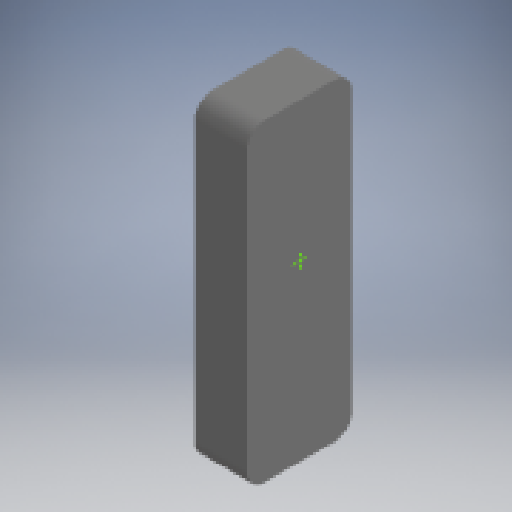
# Autodesk Inventor part: link7
Saved by Autodesk Inventor 2024.1 (Build 281209000, 209)
## iProperties
Created: 2023-09-09
Part Number: link7
Material: Aluminum 6061
Document SubType Name: Modeling
Designer: Camilo
Density: 2.7 g/cm^3
Appearance: Aluminum - Flat
Mass: 7.14896 g
Surface Area: 15.3631 cm^2
Volume: 2.64776 cm^3
Author: Camilo
Autodesk Inventor part; units mm, degrees
ref_plane "YZ Plane" through (0, 0, 0) normal (1, 0, 0) x (0, 1, 0)
ref_plane "XZ Plane" through (0, 0, 0) normal (0, 1, 0) x (-1, 0, 0)
ref_plane "XY Plane" through (0, 0, 0) normal (0, 0, 1) x (1, 0, 0)
sketch "Sketch1" plane through (0, 0, 0) normal (0, 0, 1) x (1, 0, 0)
  line L0 (0, 0) -> (0, 6)
  line L1 (0, 6) -> (-4, 6)
  line L2 (-4, 6) -> (-4, -6)
  line L3 (-4, -6) -> (0, -6)
  line L4 (0, -6) -> (0, 6)
  line L5 (-2, 6) -> (-2, -6)
  line L6 (-2, 6) -> (-2, 3)
  circle A0 centre (-2, 3) radius 1.25
  line L7 (-2, -6) -> (-2, -3)
  circle A1 centre (-2, -3) radius 1.25
  line L8 (0, 6) -> (0, 14)
  line L9 (0, 14) -> (6, 14)
  line L10 (6, 14) -> (6, -22)
  line L11 (6, -22) -> (0, -22)
  line L12 (0, -22) -> (0, 14)
  dimension "d44" = 6
  dimension "d45" = 4
  dimension "d46" = 12
  dimension "d47" = 3
  dimension "d48" = 2.5
  dimension "d49" = 3
  dimension "d50" = 2.5
  dimension "d51" = 8
  dimension "d52" = 6
  dimension "d53" = 36
  constraints: 26 end point, 4 parallel, 2 centre point, 2 coincident, 2 horizontal, 2 midpoint, 2 perpendicular, 2 point on line, 2 vertical
  measures "d44" distance of L0.start L0.end
  measures "d45" distance of L3.end L2.end
  measures "d46" distance of L2.end L1.end
  measures "d47" distance of L5.start L6.end
  measures "d48" diameter of A0
  measures "d49" distance of L5.end L7.end
  measures "d50" diameter of A1
  measures "d51" distance of L0.end L8.end
  measures "d52" distance of L10.end L11.end
  measures "d53" distance of L9.end L10.end
extrude "Extrusion8" add sketch "Sketch1" along normal mid plane 2 contours L4 L3 L5 A1 A0 L1 L0 | L5 A0 A1 L3 L2 L1
extrude "Extrusion9" add sketch "Sketch1" along normal mid plane 12 contours L0 L8 L9 L10 L11 L12 L4
fillet "Fillet1" radius 2 4 edges at (3, 14, 6) (3, 14, -6) (3, -22, 6) (3, -22, -6)
sketch "Sketch2" plane through (6, -20, -6) normal (1, 0, 0) x (0, 0, -1)
  point P0 (-6, 18)
body "Solid3"
